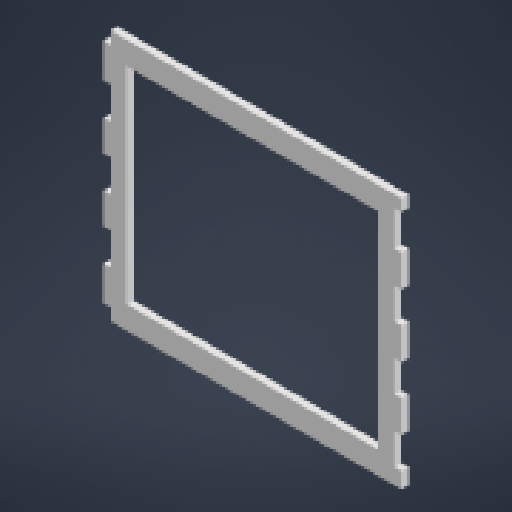
# Autodesk Inventor part: Pieza5
Saved by Autodesk Inventor 2026.1 (Build 301233020, 233B)
## iProperties
Created: 2026-05-06
Part Number: Pieza5
Material: Genérico
Document SubType Name: Modeling
Designer: OlmesTech
Density: 1 g/cm^3
Appearance: Valor por defecto
Author: OlmesTech
Autodesk Inventor part; units mm, degrees
ref_plane "YZ Plane" through (0, 0, 0) normal (1, 0, 0) x (0, 1, 0)
ref_plane "XZ Plane" through (0, 0, 0) normal (0, 1, 0) x (-1, 0, 0)
ref_plane "XY Plane" through (0, 0, 0) normal (0, 0, 1) x (1, 0, 0)
sketch "Boceto1" plane through (0, 0, 0) normal (0, 0, 1) x (1, 0, 0)
  line L0 (3, 3) -> (130, 3)
  line L1 (10, 103) -> (10, 13)
  line L2 (10, 13) -> (120, 13)
  line L3 (120, 13) -> (120, 103)
  line L4 (10, 103) -> (120, 103)
  line L5 (130, 113) -> (130, 106)
  line L6 (130, 106) -> (127, 107.7321)
  line L7 (130, 92.5) -> (127, 90.7679)
  line L8 (130, 65) -> (127, 63.2679)
  line L9 (130, 78.5) -> (127, 80.2321)
  line L10 (130, 10) -> (127, 8.2679)
  line L11 (130, 23.5) -> (127, 25.2321)
  line L12 (130, 51) -> (127, 52.7321)
  line L13 (130, 37.5) -> (127, 35.7679)
  line L14 (127, 107.7321) -> (127, 90.7679)
  line L15 (127, 80.2321) -> (127, 63.2679)
  line L16 (127, 52.7321) -> (127, 35.7679)
  line L17 (127, 25.2321) -> (127, 8.2679)
  line L18 (3, 113) -> (3, 106)
  line L19 (3, 106) -> (0, 107.7321)
  line L20 (3, 92.5) -> (0, 90.7679)
  line L21 (3, 65) -> (0, 63.2679)
  line L22 (3, 78.5) -> (0, 80.2321)
  line L23 (3, 10) -> (0, 8.2679)
  line L24 (3, 23.5) -> (0, 25.2321)
  line L25 (3, 37.5) -> (0, 35.7679)
  line L26 (3, 51) -> (0, 52.7321)
  line L27 (0, 107.7321) -> (0, 90.7679)
  line L28 (0, 80.2321) -> (0, 63.2679)
  line L29 (0, 52.7321) -> (0, 35.7679)
  line L30 (0, 25.2321) -> (0, 8.2679)
  line L31 (130, 113) -> (130, 106)
  line L32 (130, 92.5) -> (130, 85.5)
  line L33 (130, 113) -> (130, 106)
  line L34 (130, 113) -> (130, 106)
  line L35 (130, 92.5) -> (130, 78.5)
  line L36 (130, 92.5) -> (130, 78.5)
  line L37 (130, 65) -> (130, 58)
  line L38 (130, 65) -> (130, 51)
  line L39 (130, 37.5) -> (130, 23.5)
  line L40 (130, 10) -> (130, 3)
  line L41 (0, 8.2679) -> (0, 25.2321)
  line L42 (0, 35.7679) -> (0, 52.7321)
  line L43 (0, 63.2679) -> (0, 80.2321)
  line L44 (0, 90.7679) -> (0, 107.7321)
  line L45 (3, 113) -> (3, 106)
  line L46 (3, 92.5) -> (3, 85.5)
  line L47 (3, 113) -> (3, 106)
  line L48 (3, 113) -> (3, 106)
  line L49 (3, 92.5) -> (3, 78.5)
  line L50 (3, 92.5) -> (3, 78.5)
  line L51 (3, 65) -> (3, 58)
  line L52 (3, 65) -> (3, 51)
  line L53 (3, 37.5) -> (3, 23.5)
  line L54 (3, 10) -> (3, 3)
  line L55 (3, 113) -> (130, 113)
  line L56 (0, 107.7321) -> (3, 107.7321)
  line L57 (0, 92.5) -> (3, 92.5)
  line L58 (0, 78.5) -> (3, 78.5)
  line L59 (0, 65) -> (3, 65)
  line L60 (0, 51) -> (3, 51)
  line L61 (0, 37.5) -> (3, 37.5)
  line L62 (0, 23.5) -> (3, 23.5)
  line L63 (0, 8.2679) -> (3, 8.2679)
  line L64 (127, 107.7321) -> (130, 107.7321)
  line L65 (127, 92.5) -> (130, 92.5)
  line L66 (127, 78.5) -> (130, 78.5)
  line L67 (127, 65) -> (130, 65)
  line L68 (127, 51) -> (130, 51)
  line L69 (127, 37.5) -> (130, 37.5)
  line L70 (127, 23.5) -> (130, 23.5)
  line L71 (127, 10) -> (130, 10)
  line L72 (127, 8.2679) -> (130, 8.2679)
  point P0 (0, 0)
  point P1 (0, 58)
  point P2 (3, 3)
  point P3 (127, 99.25)
  dimension "d11" = 7
  dimension "d14" = 7
  dimension "d18" = 3
  dimension "d20" = 44.4641
  dimension "d21" = 7
  dimension "d22" = 65.5359
  dimension "d24" = 130
  dimension "d25" = 110
  dimension "d26" = 7
  constraints: 146 end point, 21 point on line, 12 equal length, 10 perpendicular, 6 midpoint, 6 vertical, 2 horizontal
  measures "d11" distance of L5.start L5.end
  measures "d14" distance of L18.start L18.end
  measures "d18" distance between parallel lines of L5 L14
  measures "d20" distance of L13.end L9.end
  measures "d21" distance from line of point (127, 99.25) L3
  measures "d22" distance of L24.end L20.end
  measures "d24" distance between parallel lines of L35 L27
  measures "d25" distance between parallel lines of L3 L1
  measures "d26" distance from line of point (3, 85.5) L1
extrude "Extrusión1" add sketch "Boceto1" against normal blind 3 contours L54 L23 L30 L62 L53 L61 L29 L60 L52 L51 L59 L28 L58 L49 L46 L57 L27 L19 L18 L55 L5 L64 L14 L7 L32 L35 L9 L15 L8 L37 L38 L12 L16 L13 L39 L11 L17 L72 L40 L0 | L63 L23 L54 | L72 L10 L40 | L10 L17 L71 | L17 L11 L70 | L13 L16 L69 | L16 L12 L68 | L8 L15 L67 | L15 L9 L66 | L7 L14 L65 | L56 L18 L19
